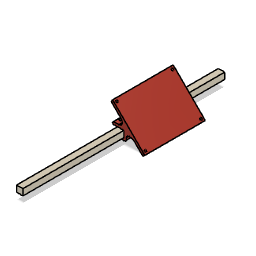
230314 Specimen mounting (Autodesk Fusion 360 design; units mm, degrees)
Autodesk Fusion 360 part; units mm, degrees
sketch "Sketch1" plane through (0, 0, 0) normal (0, 0, 1) x (1, 0, 0)
  line L0 (0, 0) -> (12.5, 0)
  line L1 (12.5, 0) -> (12.5, 12.5)
  line L2 (12.5, 12.5) -> (0, 12.5)
  line L3 (0, 12.5) -> (0, 0)
  line L4 (-15, 12.5) -> (25.5711, 12.5)
  line L5 (17.3964, -5) -> (-5, -5)
  line L6 (-15, 7.5) -> (-15, 12.5)
  line L7 (-15, -5) -> (-5, -5)
  line L8 (-5, -5) -> (-5, 7.5)
  line L9 (-5, 7.5) -> (-15, 7.5)
  line L10 (17.5, -5) -> (17.5, 7.5)
  line L11 (17.5, 7.5) -> (23.5, 7.5)
  line L12 (17.5, -4.8205) -> (17.3964, -5)
  line L13 (-15, 12.5) -> (18.5, 12.5)
  line L14 (19.5711, 18.5) -> (-15, 18.5)
  line L15 (-15, 18.5) -> (-15, 12.5)
  line L16 (12.5, 18.5) -> (-8.7132, 39.7132)
  line L17 (12.5, 18.5) -> (19.5711, 18.5) construction
  line L18 (12.5, 18.5) -> (54.9264, -23.9264)
  line L19 (-8.7132, 39.7132) -> (-5.1777, 43.2487)
  line L20 (-5.1777, 43.2487) -> (61.9975, -23.9264)
  line L21 (54.9264, -23.9264) -> (61.9975, -23.9264)
  line L22 (12.5, 18.5) -> (19.5711, 18.5) construction
  line L23 (45, 18.5) -> (72.5, 18.5) construction
  dimension "d1" = 12.5
  dimension "d2" = 12.5
  dimension "d3" = 5
  dimension "d4" = 12.5
  dimension "d5" = 15
  dimension "d10" = 5
  dimension "d11" = 5
  dimension "d12" = 5
  dimension "d13" = 5
  dimension "d15" = 6
  dimension "d16" = 135
  dimension "d17" = 30
  dimension "d18" = 45
  dimension "d19" = 60
  dimension "d20" = 5
  constraint horizontal L0
  constraint vertical L1
  constraint horizontal L2
  constraint vertical L3
  constraint coincident L0.start L3.end
  constraint horizontal L4
  constraint horizontal L5
  constraint vertical L6
  constraint horizontal L7
  constraint vertical L8
  constraint horizontal L9
  constraint coincident L5 L10.start
  constraint perpendicular L5 L10
  constraint perpendicular L10 L11
  constraint coincident L10 L12.start
  constraint horizontal L13
  constraint horizontal L14
  constraint vertical L15
  constraint horizontal L17
  constraint coincident L14 L16.start
  constraint horizontal L22
  constraint perpendicular L16 L19
  constraint parallel L18 L20
  constraint coincident L18 L11.end
  constraint coincident L20 L14.start
  constraint coincident L20 L4.end
  constraint collinear L22 L23
  constraint coincident L18 L13.end
  measures "d1" distance of L0.start L0.end
  measures "d2" distance of L0.start L2.end
  measures "d3" distance of L0 L5
  measures "d4" distance of L0.start L4
  measures "d5" distance of L0.start L6
  measures "d10" distance of L3 L8
  measures "d11" distance of L4 L9
  measures "d12" distance of L1 L10
  measures "d13" distance of L4 L11
  measures "d15" distance of L4.start L14.end
  measures "d16" angle of L16 L17
  measures "d17" distance of L16.start L16.end
  measures "d18" angle of L18 L22
  measures "d19" distance of L16.start L18.end
  measures "d20" distance of L16.end L19.end
sketch "Sketch2" plane through (0, 0, 0) normal (0, 0, 1) x (1, 0, 0)
  line L0 (0, 0) -> (-20.5, 0)
  line L1 (-12.5, 0) -> (-12.5, -12.5)
  line L2 (-20.5, -12.5) -> (0, -12.5)
  line L3 (0, -12.5) -> (0, 0)
  line L4 (-9.7844, 5) -> (-20.5, 5)
  line L5 (-20.5, -17.5) -> (2, -17.5)
  line L6 (-22.5, 3) -> (-22.5, 2)
  line L7 (-22.5, -14.5) -> (-22.5, -15.5)
  line L8 (7.1151, 5) -> (37.353, 5) construction
  line L9 (41.4129, -22.2267) -> (-22.2267, 41.4129)
  line L10 (5, -21) -> (5, -20)
  line L11 (-22.2267, 41.4129) -> (-24.348, 39.2916)
  line L12 (41.4129, -22.2267) -> (39.2916, -24.348)
  line L13 (10, -5) -> (10.4877, -5)
  line L14 (5, -14.5) -> (5, -10)
  line L15 (36.4631, -24.348) -> (21.8014, -9.6863)
  line L16 (-4.8346, 16.9497) -> (-24.348, 36.4631)
  arc A0 (-9.7844, 5) -> (-4.8346, 16.9497) centre (-9.7844, 12) ccw
  arc A1 (2, -17.5) -> (5, -14.5) centre (2, -14.5) ccw
  arc A2 (-22.5, -15.5) -> (-20.5, -17.5) centre (-20.5, -15.5) ccw
  arc A3 (-20.5, -12.5) -> (-22.5, -14.5) centre (-20.5, -14.5) ccw
  arc A4 (-22.5, 2) -> (-20.5, 0) centre (-20.5, 2) ccw
  arc A5 (-20.5, 5) -> (-22.5, 3) centre (-20.5, 3) ccw
  arc A6 (-24.348, 39.2916) -> (-24.348, 36.4631) centre (-22.9338, 37.8774) ccw
  arc A7 (36.4631, -24.348) -> (39.2916, -24.348) centre (37.8774, -22.9338) ccw
  arc A8 (10, -5) -> (5, -10) centre (10, -10) ccw
  arc A9 (21.8014, -9.6863) -> (10.4877, -5) centre (10.4877, -21) ccw
  point P0 (-25.7622, 37.8774)
  point P1 (37.8774, -25.7622)
  dimension "d21" = 12.5
  dimension "d22" = 12.5
  dimension "d23" = 5
  dimension "d24" = 5
  dimension "d25" = 10
  dimension "d26" = 135
  dimension "d29" = 90
  dimension "d30" = 5
  dimension "d31" = 5
  dimension "d32" = 7
  dimension "d33" = 3
  dimension "d34" = 2
  dimension "d35" = 2
  dimension "d36" = 45
  dimension "d37" = 5
  dimension "d38" = 16
  constraint horizontal L0
  constraint vertical L1
  constraint horizontal L2
  constraint vertical L3
  constraint coincident L0.start L3.end
  constraint horizontal L4
  constraint vertical L6
  constraint horizontal L5
  constraint coincident L1.start L0
  constraint coincident L1.end L2
  constraint collinear L6 L7
  constraint horizontal L8
  constraint coincident L8.start L15
  constraint perpendicular L5 L10
  constraint perpendicular L11 L15
  constraint perpendicular L12 L15
  constraint horizontal L13
  constraint vertical L14
  constraint collinear L15 L16
  constraint coincident L8.start L4
  constraint coincident L8.start L16
  constraint tangent L4 A0
  constraint tangent L16 A0
  constraint tangent L14 A1
  constraint tangent L5 A1
  constraint tangent L5 A2
  constraint tangent L7 A2
  constraint tangent L2 A3
  constraint tangent L7 A3
  constraint equal A2 A3
  constraint tangent L0 A4
  constraint tangent L6 A4
  constraint equal A2 A4
  constraint tangent L4 A5
  constraint tangent L6 A5
  constraint equal A2 A5
  constraint coincident P0 L16
  constraint coincident P0 L11
  constraint tangent L16 A6
  constraint tangent L11 A6
  constraint equal A2 A6
  constraint coincident P1 L12
  constraint coincident P1 L15
  constraint tangent L12 A7
  constraint tangent L15 A7
  constraint tangent L13 A8
  constraint tangent L14 A8
  constraint tangent L13 A9
  constraint tangent L15 A9
  measures "d21" distance of L0.start L1.start
  measures "d22" distance of L0.start L2.end
  measures "d23" distance of L0 L4
  measures "d24" distance of L2 L5
  measures "d25" distance of L1 L6
  measures "d26" angle of L8 L15
  measures "d29" distance of P0 P1
  measures "d30" distance of L3 L14
  measures "d31" distance of L0 L13
  measures "d32" radius of A0
  measures "d33" radius of A1
  measures "d34" radius of A2
  measures "d35" radius of A7
  measures "d36" distance of L0.start L11
  measures "d37" radius of A8
  measures "d38" radius of A9
extrude "Extrude1" add sketch "Sketch2" against normal blind 120 contours L0 L2 L3 L4 L5 L6 L7 L9 L11 L12 L13 L14 L15 L16 A0 A1 A2 A3 A4 A5 A6 A7 A8 A9 makes body 1
extrude "Extrude2" add sketch "Sketch2" along normal blind 200 and the other way blind 200 separate body contours L0 L1 L2 L3 makes body 2
sketch "Sketch3" plane through (9.5931, 9.5931, 0) normal (0.707107, 0.707107, 0) x (0, 0, -1)
  line L0 (0, 45) -> (0, -45)
  line L1 (0, -45) -> (120, -45)
  line L2 (120, -45) -> (120, 45)
  line L3 (120, 45) -> (0, 45)
  line L4 (0, -45) -> (120, -45)
  line L5 (120, -45) -> (120, -40)
  line L6 (120, -40) -> (0, -40)
  line L7 (0, -40) -> (0, -45)
  dimension "d45" = 120
  dimension "d46" = 5
  constraint horizontal L4
  constraint vertical L5
  constraint horizontal L6
  constraint vertical L7
  constraint coincident L0.end L1.start
  measures "d45" distance of L0.end L1.end
  measures "d46" distance of L0.end L6.end
sketch "Sketch4" plane through (0, -17.5, 0) normal (0, -1, 0) x (1, 0, 0)
  line L0 (2, -120) -> (2, 0)
  line L1 (2, 0) -> (-20.5, 0)
  line L2 (-20.5, 0) -> (-20.5, -120)
  circle A0 centre (-16.5, -10) radius 2.5
  circle A1 centre (-16.5, -57.5) radius 2.5
  circle A2 centre (-16.5, -105) radius 2.5
  line L3 (-20.5, -120) -> (2, -120)
  dimension "d57" = 5
  dimension "d58" = 10
  dimension "d59" = 16.5
  dimension "d62" = 0
  dimension "d63" = -95
  measures "d57" diameter of A0
  measures "d58" vertical distance of origin A0.centre
  measures "d59" horizontal distance of origin A0.centre
extrude "Extrude4" cut sketch "Sketch4" against normal blind 30 contours A0 | A1 | A2 bodies 1
sketch "Sketch5" plane through (9.5931, 9.5931, 0) normal (0.707107, 0.707107, 0) x (0, 0, -1)
  line L0 (0, 45) -> (0, -45)
  line L1 (0, -45) -> (120, -45)
  line L2 (120, -45) -> (120, 45)
  line L3 (120, 45) -> (0, 45)
  circle A0 centre (5, 40) radius 2.05
  line L4 (10, 35) -> (110, 35)
  line L5 (110, 35) -> (110, -35)
  line L6 (110, -35) -> (10, -35)
  line L7 (10, -35) -> (10, 35)
  circle A1 centre (115, 40) radius 2.05
  circle A2 centre (5, -40) radius 2.05
  circle A3 centre (115, -40) radius 2.05
  dimension "d66" = 4.1
  dimension "d67" = 100
  dimension "d68" = 70
  dimension "d69" = 10
  dimension "d70" = 5
  dimension "d71" = 5
  dimension "d74" = 110
  dimension "d75" = -80
  constraint horizontal L4
  constraint vertical L5
  constraint horizontal L6
  constraint vertical L7
  measures "d66" diameter of A0
  measures "d67" distance of L4.start L4.end
  measures "d68" distance of L4.start L6.end
  measures "d69" distance of L3 L4
  measures "d70" distance of L3 A0.centre
  measures "d71" distance of L0 A0.centre
extrude "Extrude5" cut sketch "Sketch5" against normal blind 15 contours A0 | A1 | A2 | A3 bodies 1
named bodies: "steel holder", "fence bar"
